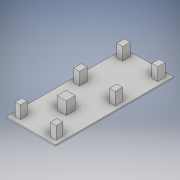
# Autodesk Inventor part: cstand
Saved by Autodesk Inventor 2019 (Build 230136000, 136)
## iProperties
Created: 2020-02-18
Part Number: cstand
Material: Generic
Document SubType Name: Modeling
Designer: Dell
Density: 1 g/cm^3
Appearance: Default
Author: Dell
Autodesk Inventor part; units mm, degrees
ref_plane "YZ Plane" through (0, 0, 0) normal (1, 0, 0) x (0, 1, 0)
ref_plane "XZ Plane" through (0, 0, 0) normal (0, 1, 0) x (-1, 0, 0)
ref_plane "XY Plane" through (0, 0, 0) normal (0, 0, 1) x (1, 0, 0)
sketch "Sketch1" plane through (0, 0, 0) normal (0, 1, 0) x (-1, 0, 0)
  line L0 (126.3491, 283.4802) -> (-143.6509, 283.4802)
  line L1 (-143.6509, 283.4802) -> (-143.6509, -366.5198)
  line L2 (-143.6509, -366.5198) -> (126.3491, -366.5198)
  line L3 (126.3491, -366.5198) -> (126.3491, 283.4802)
  point P0 (0, 0)
  dimension "d0" = 650
  dimension "d1" = 270
  constraints: 8 end point, 2 parallel, 1 horizontal, 1 perpendicular
  measures "d0" distance of L2.end L0.start
  measures "d1" distance of L1.end L2.end
extrude "Extrusion1" add sketch "Sketch1" along normal blind 7
sketch "Sketch2" plane through (0, 0, 0) normal (0, -1, 0) x (1, 0, 0)
  line L0 (-101.3766, -334.6757) -> (-65.0758, -334.6757)
  line L1 (-65.0758, -334.6757) -> (-65.0758, -293.0626)
  line L2 (-65.0758, -293.0626) -> (-101.3766, -293.0626)
  line L3 (-101.3766, -293.0626) -> (-101.3766, -334.6757)
  line L4 (-97.1426, 224.249) -> (-79.8855, 224.249)
  line L5 (-79.8855, 224.249) -> (-79.8855, 190.7676)
  line L6 (-79.8855, 190.7676) -> (-97.1426, 190.7676)
  line L7 (-97.1426, 190.7676) -> (-97.1426, 224.249)
  line L8 (-106.8404, 242.9144) -> (-83.2262, 242.9144)
  line L9 (-83.2262, 242.9144) -> (-83.2262, 210.6642)
  line L10 (-83.2262, 210.6642) -> (-106.8404, 210.6642)
  line L11 (-106.8404, 210.6642) -> (-106.8404, 242.9144)
  point P0 (0, 0)
  constraints: 24 end point, 6 parallel, 3 horizontal, 3 perpendicular
sketch "Sketch3" plane through (0, 7, 0) normal (0, 1, 0) x (1, 0, 0)
  line L0 (-102.0983, -222.5922) -> (-73.128, -222.5922)
  line L1 (-73.128, -222.5922) -> (-73.128, -260.2535)
  line L2 (-73.128, -260.2535) -> (-102.0983, -260.2535)
  line L3 (-102.0983, -260.2535) -> (-102.0983, -222.5922)
  point P0 (0, 0)
  constraints: 8 end point, 2 parallel, 1 horizontal, 1 perpendicular
extrude "Extrusion2" add sketch "Sketch3" along normal blind 70 and the other way blind 5
sketch "Sketch4" plane through (0, 7, 0) normal (0, 1, 0) x (1, 0, 0)
  line L0 (123.5415, -260.2535) -> (92.3696, -260.2535)
  line L1 (92.3696, -260.2535) -> (92.3696, -223.4411)
  line L2 (92.3696, -223.4411) -> (123.5415, -223.4411)
  line L3 (123.5415, -223.4411) -> (123.5415, -260.2535)
  point P0 (0, 0)
  constraints: 8 end point, 2 parallel, 1 horizontal, 1 perpendicular
extrude "Extrusion3" add sketch "Sketch4" along normal blind 70
sketch "Sketch5" plane through (0, 7, 0) normal (0, 1, 0) x (1, 0, 0)
  line L0 (123.5415, 64.5703) -> (92.3696, 64.5703)
  line L1 (92.3696, 64.5703) -> (92.3696, 104.6485)
  line L2 (92.3696, 104.6485) -> (123.5415, 104.6485)
  line L3 (123.5415, 104.6485) -> (123.5415, 64.5703)
  point P0 (0, 0)
  constraints: 8 end point, 2 parallel, 1 horizontal, 1 perpendicular
extrude "Extrusion4" add sketch "Sketch5" along normal blind 70
sketch "Sketch6" plane through (0, 7, 0) normal (0, 1, 0) x (1, 0, 0)
  line L0 (-70.3594, 62.7891) -> (-102.4219, 62.7891)
  line L1 (-102.4219, 62.7891) -> (-102.4219, 105.5391)
  line L2 (-102.4219, 105.5391) -> (-70.3594, 105.5391)
  line L3 (-70.3594, 105.5391) -> (-70.3594, 62.7891)
  point P0 (0, 0)
  constraints: 8 end point, 2 parallel, 1 horizontal, 1 perpendicular
extrude "Extrusion5" add sketch "Sketch6" along normal blind 70
sketch "Sketch7" plane through (0, 7, 0) normal (0, 1, 0) x (1, 0, 0)
  line L0 (-102.4219, 342.1053) -> (-70.3594, 342.1053)
  line L1 (-70.3594, 342.1053) -> (-70.3594, 300.246)
  line L2 (-70.3594, 300.246) -> (-102.4219, 300.246)
  line L3 (-102.4219, 300.246) -> (-102.4219, 342.1053)
  point P0 (0, 0)
  constraints: 8 end point, 2 parallel, 1 horizontal, 1 perpendicular
extrude "Extrusion6" add sketch "Sketch7" along normal blind 70
sketch "Sketch8" plane through (0, 7, 0) normal (0, 1, 0) x (1, 0, 0)
  line L0 (123.5415, 300.5975) -> (89.9566, 300.5975)
  line L1 (89.9566, 300.5975) -> (89.9566, 340.6771)
  line L2 (89.9566, 340.6771) -> (123.5415, 340.6771)
  line L3 (123.5415, 340.6771) -> (123.5415, 300.5975)
  point P0 (0, 0)
  constraints: 8 end point, 2 parallel, 1 horizontal, 1 perpendicular
extrude "Extrusion7" add sketch "Sketch8" along normal blind 70
sketch "Sketch9" plane through (0, 7, 0) normal (0, 1, 0) x (1, 0, 0)
  line L0 (33.3984, -64.125) -> (-17.3672, -64.125)
  line L1 (-17.3672, -64.125) -> (-17.3672, -114)
  line L2 (-17.3672, -114) -> (33.3984, -114)
  line L3 (33.3984, -114) -> (33.3984, -64.125)
  point P0 (0, 0)
  constraints: 8 end point, 2 parallel, 1 horizontal, 1 perpendicular
extrude "Extrusion8" add sketch "Sketch9" along normal blind 70
body "Solid1"
